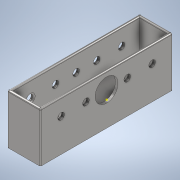
# Autodesk Inventor part: gear holder
Saved by Autodesk Inventor 2022 (Build 260153070, 153G)
## iProperties
Created: 2021-06-28
Part Number: gear holder
Material: Stainless Steel
Document SubType Name: Modeling
Designer: AKASH ARYAN
Density: 8 g/cm^3
Appearance: Semi-Polished
Author: AKASH ARYAN
Autodesk Inventor part; units mm, degrees
ref_plane "YZ Plane" through (0, 0, 0) normal (1, 0, 0) x (0, 1, 0)
ref_plane "XZ Plane" through (0, 0, 0) normal (0, 1, 0) x (-1, 0, 0)
ref_plane "XY Plane" through (0, 0, 0) normal (0, 0, 1) x (1, 0, 0)
sketch "Sketch1" plane through (0, 0, 0) normal (1, 0, 0) x (0, 1, 0)
  line L0 (38.1, 101.6) -> (-38.1, 101.6)
  line L1 (-38.1, 101.6) -> (-38.1, -101.6)
  line L2 (-38.1, -101.6) -> (38.1, -101.6)
  line L3 (38.1, -101.6) -> (38.1, 101.6)
  line L4 (38.1, 101.6) -> (-38.1, -101.6) construction
  line L5 (-38.1, 101.6) -> (38.1, -101.6) construction
  point P0 (0, 0)
  dimension "d0" = 76.2
  dimension "d1" = 203.2
  constraints: 12 end point, 2 midpoint, 2 parallel, 1 horizontal, 1 perpendicular
  measures "d0" distance of L2.end L1.end
  measures "d1" distance of L1.end L0.end
extrude "Extrusion1" add sketch "Sketch1" along normal mid plane 50.8
sketch "Sketch2" plane through (-25.4, 38.1, 101.6) normal (0, 1, 0) x (1, 0, 0)
  line L0 (4, 199.2) -> (46.8, 199.2)
  line L1 (46.8, 199.2) -> (46.8, 4)
  line L2 (46.8, 4) -> (4, 4)
  line L3 (4, 4) -> (4, 199.2)
  line L4 (4, 199.2) -> (46.8, 4) construction
  line L5 (46.8, 199.2) -> (4, 4) construction
  line L6 (0, 0) -> (0, 203.2) projected
  line L7 (0, 0) -> (50.8, 0) projected
  point P0 (25.4, 101.6)
  dimension "d4" = 4
  dimension "d5" = 4
  constraints: 12 end point, 2 midpoint, 2 parallel, 1 horizontal, 1 perpendicular
  measures "d4" distance between parallel lines of L6 L3
  measures "d5" distance between parallel lines of L7 L2
extrude "Extrusion2" cut sketch "Sketch2" against normal blind 47.8
sketch "Sketch5" plane through (-25.4, -38.1, -101.6) normal (0, -1, 0) x (1, 0, 0)
  circle A0 centre (25.4, 152.4) radius 2
  circle A1 centre (25.4, 177.8) radius 2
  circle A2 centre (25.4, 50.8) radius 2
  circle A3 centre (25.4, 25.4) radius 2
  line L0 (50.8, 203.2) -> (0, 203.2) projected
  line L1 (0, 0) -> (50.8, 0) projected
  line L2 (50.8, 203.2) -> (50.8, 0) projected
  point P0 (25.4, 101.6)
  dimension "d33" = 4
  dimension "d34" = 4
  dimension "d35" = 4
  dimension "d36" = 4
  dimension "d37" = 25.4
  dimension "d38" = 25.4
  dimension "d39" = 50.8
  dimension "d40" = 50.8
  dimension "d41" = 25.4
  dimension "d42" = 25.4
  dimension "d43" = 25.4
  dimension "d44" = 25.4
  constraints: 4 centre point
  measures "d33" diameter of A0
  measures "d34" diameter of A1
  measures "d35" diameter of A2
  measures "d36" diameter of A3
  measures "d37" distance from line of L0 A1.centre
  measures "d38" distance from line of A3.centre L1
  measures "d39" distance from line of L0 A0.centre
  measures "d40" distance from line of L1 A2.centre
  measures "d41" distance from line of L2 A2.centre
  measures "d42" distance from line of L2 A3.centre
  measures "d43" distance from line of L2 A1.centre
  measures "d44" distance from line of L2 A0.centre
extrude "Extrusion5" cut sketch "Sketch5" against normal through all
sketch "Sketch6" plane through (25.4, 0, 0) normal (1, 0, 0) x (0, 0, -1)
  point P0 (0, 0)
sketch "Sketch7" plane through (25.4, 0, 0) normal (1, 0, 0) x (0, 0, -1)
  point P0 (0, 0)
sketch "Sketch8" plane through (25.4, 0, 0) normal (1, 0, 0) x (0, 0, -1)
  circle A0 centre (-69.85, 12.7) radius 5
  circle A1 centre (-31.75, 12.7) radius 5
  circle A2 centre (31.75, 12.7) radius 5
  circle A3 centre (69.85, 12.7) radius 5
  line L0 (-101.6, 38.1) -> (-101.6, -38.1)
  line L1 (101.6, -38.1) -> (101.6, 38.1)
  line L2 (101.6, 38.1) -> (-101.6, 38.1) projected
  point P0 (0, 0)
  dimension "d47" = 10
  dimension "d48" = 10
  dimension "d49" = 10
  dimension "d50" = 10
  dimension "d51" = 31.75
  dimension "d52" = 69.85
  dimension "d53" = 31.75
  dimension "d54" = 69.85
  dimension "d55" = 25.4
  dimension "d56" = 25.4
  dimension "d57" = 25.4
  dimension "d58" = 25.4
  constraints: 4 centre point, 4 end point
  measures "d47" diameter of A0
  measures "d48" diameter of A1
  measures "d49" diameter of A2
  measures "d50" diameter of A3
  measures "d51" distance from line of L0 A0.centre
  measures "d52" distance from line of L0 A1.centre
  measures "d53" distance from line of L1 A3.centre
  measures "d54" distance from line of L1 A2.centre
  measures "d55" distance from line of L2 A0.centre
  measures "d56" distance from line of A1.centre L2
  measures "d57" distance from line of A2.centre L2
  measures "d58" distance from line of A3.centre L2
sketch "Sketch9" plane through (25.4, 0, 0) normal (1, 0, 0) x (0, 0, -1)
  point P0 (0, 0)
sketch "Sketch10" plane through (25.4, 0, 0) normal (1, 0, 0) x (0, 0, -1)
  point P0 (0, 0)
extrude "Extrusion6" cut sketch "Sketch8" against normal through all
fillet "Fillet1" radius 2 13 edges at (0, 38.1, 101.6) (0, 38.1, 97.6) (-21.4, 12.7, 74.85) (25.4, 38.1, 0) (21.4, 38.1, 0) (-21.4, 38.1, 0) (-25.4, 38.1, 0) (0, 38.1, -97.6) (0, 38.1, -101.6) (25.4, 0, 101.6) (-25.4, 0, 101.6) (25.4, 0, -101.6) (-25.4, 0, -101.6)
sketch "Sketch11" plane through (0, 0, 0) normal (0, 1, 0) x (-1, 0, 0)
  point P0 (0, 0)
sketch "Sketch12" plane through (0, 0, 0) normal (0, 1, 0) x (-1, 0, 0)
  point P0 (0, 0)
sketch "Sketch13" plane through (-25.4, 0, 0) normal (-1, 0, 0) x (0, 0, 1)
  circle A0 centre (0, 12.7) radius 5
  line L0 (-99.6, -38.1) -> (99.6, -38.1) projected
  point P0 (0, 0)
  dimension "d62" = 10
  dimension "d63" = 50.8
  constraints: 1 centre point
  measures "d62" diameter of A0
  measures "d63" distance from line of L0 A0.centre
extrude "Extrusion7" cut sketch "Sketch13" against normal blind 4
sketch "Sketch14" plane through (25.4, 0, 0) normal (1, 0, 0) x (0, 0, -1)
  circle A0 centre (0, 12.7) radius 17.5
  line L0 (-99.6, 36.1) -> (99.6, 36.1) projected
  point P0 (0, 0)
  dimension "d66" = 35
  dimension "d69" = 23.4
  constraints: 1 centre point
  measures "d66" diameter of A0
  measures "d69" distance from line of A0.centre L0
extrude "Extrusion8" cut sketch "Sketch14" against normal blind 4
sketch "Sketch15" plane through (25.4, 0, 0) normal (1, 0, 0) x (0, 0, -1)
  point P0 (0, 0)
body "Solid1"
